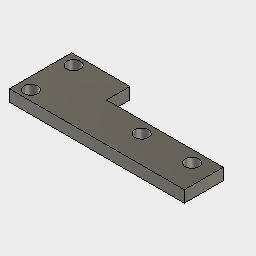
bart x ensstop bracket plain swtich v4 (Autodesk Fusion 360 design; units mm, degrees)
Autodesk Fusion 360 part; units mm, degrees
sketch "Sketch1" plane through (0, 0, 0) normal (0, 0, 1) x (1, 0, 0)
  line L0 (0, 0) -> (45, 0)
  line L1 (45, 0) -> (45, 10)
  line L2 (15, 16) -> (0, 16)
  line L3 (0, 16) -> (0, 0)
  line L4 (0, 8) -> (3, 8)
  line L5 (3, 8) -> (3, 13.5)
  line L6 (3, 13.5) -> (3, 2.5)
  circle A0 centre (3, 13.5) radius 1.75
  circle A1 centre (3, 2.5) radius 1.75
  line L7 (0, 16) -> (15, 16)
  line L8 (15, 16) -> (15, 10)
  line L9 (15, 16) -> (21, 16) construction
  line L10 (15, 10) -> (45, 10)
  line L11 (45, 10) -> (45, 7)
  line L12 (45, 7) -> (40, 7)
  line L13 (45, 7) -> (50, 7) construction
  line L14 (40, 7) -> (40, 10)
  line L15 (27, 10) -> (27, 4.4061)
  line L16 (40, 7) -> (20.1123, 7)
  circle A2 centre (27, 7) radius 1.75
  circle A3 centre (40, 7) radius 1.75
  dimension "d1" = 45
  dimension "d2" = 16
  dimension "d3" = 3
  dimension "d4" = 5.5
  dimension "d5" = 11
  dimension "d6" = 3.5
  dimension "d7" = 3.5
  dimension "d8" = 15
  dimension "d9" = 90
  dimension "d10" = 6
  dimension "d11" = 3
  dimension "d12" = 180
  dimension "d13" = 5
  dimension "d15" = 3.5
  dimension "d16" = 3.5
  constraint horizontal L0
  constraint vertical L1
  constraint horizontal L2
  constraint vertical L3
  constraint midpoint L3
  constraint perpendicular L3 L4
  constraint perpendicular L4 L5
  constraint perpendicular L4 L6
  constraint horizontal L9
  constraint perpendicular L1 L10
  constraint perpendicular L10 L11
  constraint horizontal L13
  constraint perpendicular L10 L14
  constraint perpendicular L10 L15
  constraint perpendicular L15 L16
  constraint coincident L10
  constraint coincident L16
  constraint coincident L15
  measures "d6" diameter of A0
  measures "d7" diameter of A1
  measures "d9" angle of L8 L9
  measures "d12" angle of L12 L13
  measures "d15" diameter of A2
  measures "d16" diameter of A3
extrude "Extrude1" add sketch "Sketch1" along normal blind 3 contours L0 L1 L2 L3 L7 L8 L10 L12 L15 L16 A2 A3 | L1 L10 L11 L12 L14 A3 | L10 L14 L15 L16 A2 A3
